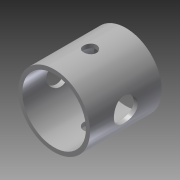
# Autodesk Inventor part: GE-13026-01
Saved by Autodesk Inventor 2013 (Build 170138000, 138)
## iProperties
Created: 2013-01-06
Part Number: GE-13026-01
Material: Steel
Document SubType Name: Modeling
Designer: Phillip
Density: 1 g/cm^3
Author: Phillip
Autodesk Inventor part; units mm, degrees
ref_plane "XY Plane" through (0, 0, 0) normal (0, 0, 1) x (1, 0, 0)
sketch "Sketch1" plane through (0, 0, 0) normal (0, 0, 1) x (1, 0, 0)
  circle A0 centre (0, 0) radius 19.05
  circle A1 centre (0, 0) radius 16.891
  dimension "d0" = 38.1
  dimension "d2" = 33.782
  constraints: 2 centre point, 2 coincident
  measures "d0" diameter of A0
  measures "d2" diameter of A1
extrude "Extrusion1" add sketch "Sketch1" against normal blind 38.1
ref_plane "Work Plane1" through (19.05, 0, 0) normal (1, 0, 0) x (0, 1, 0)
sketch "Sketch2" plane through (19.05, 0, 0) normal (1, 0, 0) x (0, 1, 0)
  line L0 (19.05, 0) -> (19.05, -38.1) projected
  point P0 (0, 0)
  point P1 (0, -19.05)
  point P2 (19.05, -19.05)
  constraints: 1 horizontal alignment, 1 midpoint, 1 vertical alignment
hole "Hole1" at (19.05, 0, -19.05) direction (-1, 0, 0) diameter 12.7 end through all
ref_plane "Work Plane2" through (0, 19.05, 0) normal (0, 1, 0) x (-1, 0, 0)
sketch "Sketch3" plane through (0, 19.05, 0) normal (0, 1, 0) x (-1, 0, 0)
  line L0 (19.05, 0) -> (19.05, -38.1) projected
  line L1 (-19.05, 0) -> (19.05, 0) projected
  point P0 (0, 0)
  point P1 (0, -19.05)
  point P2 (0, 0)
  point P3 (19.05, -19.05)
  constraints: 2 midpoint, 1 horizontal alignment, 1 vertical alignment
hole "Hole2" at (0, 19.05, -19.05) direction (0, -1, 0) diameter 6.858 end through all
body "Solid1"
